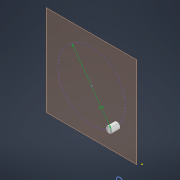
# Autodesk Inventor part: Clemma_CPY
Saved by Autodesk Inventor 2022 (Build 260153070, 153G)
## iProperties
Created: 2021-11-19
Part Number: Clemma_CPY
Material: Типовые
Document SubType Name: Modeling
Designer: kalugin_a
Density: 1 g/cm^3
Appearance: По умолчанию
Author: kalugin_a
Autodesk Inventor part; units mm, degrees
ref_plane "YZ Plane" through (0, 0, 0) normal (1, 0, 0) x (0, 1, 0)
ref_plane "XZ Plane" through (0, 0, 0) normal (0, 1, 0) x (-1, 0, 0)
ref_plane "XY Plane" through (0, 0, 0) normal (0, 0, 1) x (1, 0, 0)
sketch "Эскиз1" plane through (0, 0, 0) normal (0, 0, 1) x (1, 0, 0)
  circle A0 centre (-31.2403, 27.0306) radius 4
  line L0 (-31.9005, 24.3212) -> (-30.5802, 24.3212)
  line L1 (-30.5802, 24.3212) -> (-30.5802, 29.74)
  line L2 (-30.5802, 29.74) -> (-31.9005, 29.74)
  line L3 (-31.9005, 29.74) -> (-31.9005, 24.3212)
  line L4 (-31.9005, 24.3212) -> (-30.5802, 29.74) construction
  line L5 (-30.5802, 24.3212) -> (-31.9005, 29.74) construction
  point P0 (0, 0)
  dimension "d0" = 8
  constraints: 12 end point, 2 midpoint, 2 parallel, 1 centre point, 1 horizontal, 1 perpendicular
  measures "d0" diameter of A0
extrude "Выдавливание1" add sketch "Эскиз1" along normal blind 10
ref_plane "РабПлоскость1" through (-63.6305, 53.4641, -0.3717) normal (0, 0, 1) x (1, 0, 0)
sketch "Эскиз2" plane through (-63.6305, 53.4641, -0.3717) normal (0, 0, 1) x (1, 0, 0)
  circle A0 centre (0, 0) radius 42.5 construction
  point P0 (63.6305, -53.4641)
  dimension "d3" = 85
  constraints: 1 centre point
  measures "d3" diameter of A0
